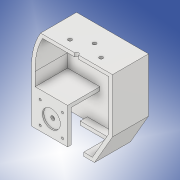
# Autodesk Inventor part: FA001
Saved by Autodesk Inventor 2017 (Build 210142000, 142)
## iProperties
Created: 2017-06-14
Part Number: FA001
Material: ABS Plastic
Document SubType Name: Modeling
Designer: zallen
Density: 1.06 g/cm^3
Appearance: CR White
Author: zallen
Autodesk Inventor part; units mm, degrees
ref_plane "YZ Plane" through (0, 0, 0) normal (1, 0, 0) x (0, 1, 0)
ref_plane "XZ Plane" through (0, 0, 0) normal (0, 1, 0) x (-1, 0, 0)
ref_plane "XY Plane" through (0, 0, 0) normal (0, 0, 1) x (1, 0, 0)
sketch "Sketch1" plane through (0, 0, 0) normal (0, 0, 1) x (1, 0, 0)
  line L0 (0, 0) -> (100, 0)
  line L1 (100, 0) -> (100, -75)
  line L2 (100, -75) -> (75, -118.3013)
  line L3 (-12.5, -50) -> (-12.5, -118.3013)
  arc A0 (0, 0) -> (-12.5, -50) centre (77.4072, -45.9143) ccw
  line L4 (-12.5, -118.3013) -> (75, -118.3013)
  dimension "d0" = 100
  dimension "d1" = 75
  dimension "d2" = 50
  dimension "d3" = 150
  dimension "d4" = 12.5
  dimension "d5" = 50
  dimension "d6" = 90
  constraints: 10 end point, 2 horizontal, 2 point on circle, 1 centre point, 1 horizontal alignment, 1 perpendicular, 1 vertical
  measures "d0" distance of L0.start L0.end
  measures "d1" distance of L0.end L1.end
  measures "d2" distance of L1.end L2.end
  measures "d3" angle of L1 L2
  measures "d4" horizontal distance of L0.start L3.start
  measures "d5" vertical distance of L0.start L3.start
  measures "d6" radius of A0
extrude "Extrusion1" add sketch "Sketch1" along normal blind 50
sketch "Sketch2" plane through (0, 0, 50) normal (0, 0, 1) x (1, 0, 0)
  line L0 (100, 0) -> (0, 0) projected
  arc A0 (0, 0) -> (-12.5, -50) centre (77.4072, -45.9143) ccw projected
  line L1 (-12.5, -50) -> (-12.5, -118.3013) projected
  line L2 (-12.5, -118.3013) -> (75, -118.3013) projected
  line L3 (75, -118.3013) -> (100, -75) projected
  line L4 (100, -75) -> (100, 0) projected
  arc A1 (2.902, -5) -> (-7.5, -49.8848) centre (77.4072, -45.9143) ccw
  line L5 (2.902, -5) -> (95, -5)
  line L6 (95, -5) -> (95, -73.6603)
  line L7 (95, -73.6603) -> (72.1132, -113.3013)
  line L8 (72.1132, -113.3013) -> (-7.5, -113.3013)
  line L9 (-7.5, -113.3013) -> (-7.5, -49.8848)
  dimension "d9" = 5
  constraints: 10 end point, 2 point on circle, 1 centre point, 5 other
  measures "d9" radial gap between concentric circles of A0 A1
extrude "Extrusion2" cut sketch "Sketch2" against normal blind 45 contours L5 L6 L7 L8 L9 A1
sketch "Sketch3" plane through (0, 0, 50) normal (0, 0, 1) x (1, 0, 0)
  line L0 (72.1132, -113.3013) -> (-7.5, -113.3013) projected
  line L1 (-12.5, -118.3013) -> (75, -118.3013) projected
  line L2 (-7.5, -113.3013) -> (60, -113.3013)
  line L3 (60, -113.3013) -> (60, -118.3013)
  line L4 (60, -118.3013) -> (-7.5, -118.3013)
  line L5 (-7.5, -118.3013) -> (-7.5, -113.3013)
  point P0 (0, 0)
  dimension "d13" = 15
  constraints: 8 end point, 2 parallel, 1 horizontal, 1 perpendicular, 1 point on line
  measures "d13" distance from line of L1.end L3
extrude "Extrusion3" cut sketch "Sketch3" against normal blind 45
sketch "Sketch4" plane through (0, 0, 0) normal (0, 1, 0) x (1, 0, 0)
  circle A0 centre (50, -50) radius 2.75
  line L0 (100, -50) -> (0, -50) projected
  point P0 (0, 0)
  dimension "d16" = 5.5
  constraints: 1 centre point, 1 coincident, 1 midpoint
  measures "d16" diameter of A0
extrude "Extrusion4" cut sketch "Sketch4" against normal through all
sketch "Sketch5" plane through (0, 0, 0) normal (0, 1, 0) x (1, 0, 0)
  arc A0 (52.75, -50) -> (47.25, -50) centre (50, -50) ccw projected
  circle A1 centre (50, -50) radius 25 construction
  circle A2 centre (50, -25) radius 2.5
  circle A3 centre (28.3494, -37.5) radius 2.5
  circle A4 centre (28.3494, -62.5) radius 2.5
  circle A5 centre (50, -75) radius 2.5
  circle A6 centre (71.6506, -62.5) radius 2.5
  circle A7 centre (71.6506, -37.5) radius 2.5
  point P0 (0, 0)
  dimension "d20" = 50
  dimension "d21" = 5
  dimension "d24" = 360
  constraints: 6 centre point, 2 vertical alignment, 1 coincident, 15 other
  measures "d21" diameter of A2
extrude "Extrusion5" cut sketch "Sketch5" against normal blind 5 contours A2 | A3 | A7
sketch "Sketch6" plane through (0, 0, 50) normal (0, 0, 1) x (1, 0, 0)
  line L0 (75, -118.3013) -> (-12.5, -118.3013) projected
  line L1 (-7.5, -118.3013) -> (37.5, -118.3013)
  line L2 (37.5, -118.3013) -> (37.5, -73.3013)
  line L3 (37.5, -73.3013) -> (-7.5, -73.3013)
  line L4 (-7.5, -73.3013) -> (-7.5, -118.3013)
  circle A0 centre (15, -95.8013) radius 2.75
  line L5 (-0.5, -111.3013) -> (30.5, -111.3013) construction
  line L6 (30.5, -111.3013) -> (30.5, -80.3013) construction
  line L7 (30.5, -80.3013) -> (-0.5, -80.3013) construction
  line L8 (-0.5, -80.3013) -> (-0.5, -111.3013) construction
  line L9 (-0.5, -111.3013) -> (30.5, -80.3013) construction
  line L10 (30.5, -111.3013) -> (-0.5, -80.3013) construction
  circle A1 centre (30.5, -80.3013) radius 1.5
  circle A2 centre (-0.5, -80.3013) radius 1.5
  circle A3 centre (-0.5, -111.3013) radius 1.5
  circle A4 centre (30.5, -111.3013) radius 1.5
  point P0 (0, 0)
  point P1 (15, -73.3013)
  point P2 (37.5, -95.8013)
  dimension "d29" = 45
  dimension "d30" = 45
  dimension "d31" = 5.5
  dimension "d32" = 31
  dimension "d33" = 31
  dimension "d34" = 3
  dimension "d35" = 3
  dimension "d36" = 3
  dimension "d37" = 3
  constraints: 20 end point, 6 midpoint, 5 centre point, 4 coincident, 4 parallel, 2 horizontal, 2 perpendicular, 1 horizontal alignment, 1 vertical alignment
  measures "d29" distance of L1.end L2.end
  measures "d30" distance of L2.end L3.end
  measures "d31" diameter of A0
  measures "d32" distance of L7.end L6.end
  measures "d33" distance of L6.end L5.end
  measures "d34" diameter of A1
  measures "d35" diameter of A2
  measures "d36" diameter of A3
  measures "d37" diameter of A4
extrude "Extrusion6" add sketch "Sketch6" against normal blind 5
sketch "Sketch7" plane through (0, 0, 50) normal (0, 0, 1) x (1, 0, 0)
  circle A0 centre (15, -95.8013) radius 2.75 projected
  circle A1 centre (15, -95.8013) radius 12.5
  point P0 (0, 0)
  dimension "d40" = 25
  constraints: 1 centre point, 1 coincident
  measures "d40" diameter of A1
extrude "Extrusion7" cut sketch "Sketch7" against normal blind 2
sketch "Sketch8" plane through (-7.5, -73.3013, 50) normal (0, 1, 0) x (1, 0, 0)
  line L0 (45, 0) -> (45, 5) projected
  line L1 (82.5, 50) -> (-5, 50) projected
  line L2 (45, 0) -> (-5, 0)
  line L3 (-5, 0) -> (-5, 50)
  line L4 (-5, 50) -> (45, 50)
  line L5 (45, 50) -> (45, 0)
  point P0 (7.5, 50)
  constraints: 8 end point, 2 parallel, 1 horizontal, 1 perpendicular
extrude "Extrusion8" add sketch "Sketch8" along normal blind 5
sketch "Sketch10" plane through (-12.5, -118.3013, 0) normal (0, -1, 0) x (1, 0, 0)
  line L0 (87.5, 0) -> (87.5, 50) projected
  line L1 (87.5, 0) -> (0, 0) projected
  line L2 (87.5, 0) -> (32.5, 0)
  line L3 (32.5, 0) -> (32.5, 15)
  line L4 (32.5, 15) -> (87.5, 15)
  line L5 (87.5, 15) -> (87.5, 0)
  line L6 (0, 0) -> (0, 50) projected
  point P0 (12.5, 0)
  dimension "d49" = 15
  dimension "d50" = 32.5
  constraints: 8 end point, 2 parallel, 1 horizontal, 1 perpendicular
  measures "d49" distance of L2.end L3.end
  measures "d50" distance between parallel lines of L6 L3
extrude "Extrusion10" add sketch "Sketch10" against normal blind 5
body "Solid1"
